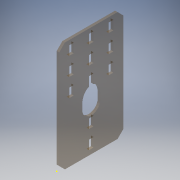
# Autodesk Inventor part: Sleigh
Saved by Autodesk Inventor 2019 (Build 230136000, 136)
## iProperties
Created: 2019-01-14
Part Number: Sleigh
Material: Polycarbonate, Smoke
Document SubType Name: Modeling
Designer: nxgam
Density: 1.2 g/cm^3
Appearance: Polycarbonate - Smoked
Author: nxgam
Autodesk Inventor part; units mm, degrees
ref_plane "YZ Plane" through (0, 0, 0) normal (1, 0, 0) x (0, 1, 0)
ref_plane "XZ Plane" through (0, 0, 0) normal (0, 1, 0) x (-1, 0, 0)
ref_plane "XY Plane" through (0, 0, 0) normal (0, 0, 1) x (1, 0, 0)
sketch "Sketch1" plane through (0, 0, 0) normal (1, 0, 0) x (0, 1, 0)
  line L0 (0, 0) -> (121.92, 0)
  line L1 (121.92, 0) -> (121.92, -71.12)
  line L2 (121.92, -71.12) -> (0, -71.12)
  line L3 (0, -71.12) -> (0, 0)
  dimension "d0" = 121.92
  dimension "d1" = 71.12
  constraints: 8 end point, 2 parallel, 1 horizontal, 1 perpendicular
  measures "d0" distance of L1.end L2.end
  measures "d1" distance of L0.end L1.end
extrude "Extrusion1" add sketch "Sketch1" along normal blind 2.794
sketch "Sketch2" plane through (2.794, 0, 0) normal (1, 0, 0) x (0, 0, -1)
  line L0 (0, 121.92) -> (0, 0) projected
  line L1 (0, 0) -> (71.12, 0) projected
  line L2 (71.12, 0) -> (71.12, 121.92) projected
  line L3 (71.12, 121.92) -> (0, 121.92) projected
  line L4 (71.12, 121.92) -> (0, 121.92) construction
  line L5 (35.56, 121.92) -> (35.56, 0) construction
  line L6 (33.02, 5.08) -> (38.1, 5.08)
  line L7 (38.1, 5.08) -> (38.1, 15.24)
  line L8 (38.1, 15.24) -> (33.02, 15.24)
  line L9 (33.02, 15.24) -> (33.02, 5.08)
  line L10 (33.02, 25.4) -> (38.1, 25.4)
  line L11 (38.1, 25.4) -> (38.1, 35.56)
  line L12 (38.1, 35.56) -> (33.02, 35.56)
  line L13 (33.02, 35.56) -> (33.02, 25.4)
  line L14 (33.02, 45.72) -> (38.1, 45.72)
  line L15 (38.1, 45.72) -> (38.1, 55.88)
  line L16 (38.1, 55.88) -> (33.02, 55.88)
  line L17 (33.02, 55.88) -> (33.02, 45.72)
  line L18 (33.02, 66.04) -> (38.1, 66.04)
  line L19 (38.1, 66.04) -> (38.1, 76.2)
  line L20 (38.1, 76.2) -> (33.02, 76.2)
  line L21 (33.02, 76.2) -> (33.02, 66.04)
  line L22 (33.02, 86.36) -> (38.1, 86.36)
  line L23 (38.1, 86.36) -> (38.1, 96.52)
  line L24 (38.1, 96.52) -> (33.02, 96.52)
  line L25 (33.02, 96.52) -> (33.02, 86.36)
  line L26 (33.02, 106.68) -> (38.1, 106.68)
  line L27 (38.1, 106.68) -> (38.1, 116.84)
  line L28 (38.1, 116.84) -> (33.02, 116.84)
  line L29 (33.02, 116.84) -> (33.02, 106.68)
  line L30 (11.049, 86.36) -> (16.129, 86.36)
  line L31 (16.129, 86.36) -> (16.129, 96.52)
  line L32 (11.049, 96.52) -> (11.049, 86.36)
  line L33 (16.129, 96.52) -> (11.049, 96.52)
  line L34 (11.049, 106.68) -> (16.129, 106.68)
  line L35 (11.049, 116.84) -> (11.049, 106.68)
  line L36 (16.129, 106.68) -> (16.129, 116.84)
  line L37 (16.129, 116.84) -> (11.049, 116.84)
  line L38 (11.049, 66.04) -> (16.129, 66.04)
  line L39 (11.049, 76.2) -> (11.049, 66.04)
  line L40 (16.129, 66.04) -> (16.129, 76.2)
  line L41 (16.129, 76.2) -> (11.049, 76.2)
  line L42 (54.991, 86.36) -> (60.071, 86.36)
  line L43 (60.071, 86.36) -> (60.071, 96.52)
  line L44 (54.991, 96.52) -> (54.991, 86.36)
  line L45 (60.071, 96.52) -> (54.991, 96.52)
  line L46 (54.991, 106.68) -> (60.071, 106.68)
  line L47 (54.991, 116.84) -> (54.991, 106.68)
  line L48 (60.071, 106.68) -> (60.071, 116.84)
  line L49 (60.071, 116.84) -> (54.991, 116.84)
  line L50 (54.991, 66.04) -> (60.071, 66.04)
  line L51 (54.991, 76.2) -> (54.991, 66.04)
  line L52 (60.071, 66.04) -> (60.071, 76.2)
  line L53 (60.071, 76.2) -> (54.991, 76.2)
  line L54 (33.02, 86.36) -> (38.1, 86.36)
  line L55 (38.1, 86.36) -> (38.1, 96.52)
  line L56 (33.02, 96.52) -> (33.02, 86.36)
  line L57 (38.1, 96.52) -> (33.02, 96.52)
  line L58 (33.02, 106.68) -> (38.1, 106.68)
  line L59 (33.02, 116.84) -> (33.02, 106.68)
  line L60 (38.1, 106.68) -> (38.1, 116.84)
  line L61 (38.1, 116.84) -> (33.02, 116.84)
  line L62 (33.02, 66.04) -> (38.1, 66.04)
  line L63 (33.02, 76.2) -> (33.02, 66.04)
  line L64 (38.1, 66.04) -> (38.1, 76.2)
  line L65 (38.1, 76.2) -> (33.02, 76.2)
  point P0 (35.56, 15.24)
  point P1 (35.56, 35.56)
  point P2 (35.56, 55.88)
  point P3 (35.56, 76.2)
  point P4 (35.56, 96.52)
  point P5 (35.56, 116.84)
  point P6 (13.589, 96.52)
  point P7 (13.589, 116.84)
  point P8 (13.589, 76.2)
  point P9 (57.531, 96.52)
  point P10 (57.531, 116.84)
  point P11 (57.531, 76.2)
  point P12 (35.56, 96.52)
  point P13 (35.56, 116.84)
  point P14 (35.56, 76.2)
  dimension "d4" = 5.08
  dimension "d5" = 10.16
  dimension "d6" = 5.08
  dimension "d9" = 20.32
  dimension "d18" = 21.971
  dimension "d21" = 21.971
  constraints: 122 end point, 3 horizontal, 3 midpoint, 2 parallel, 1 perpendicular, 1 point on line, 1 vertical, 126 other
  measures "d4" distance of L7.end L8.end
  measures "d5" distance of L6.end L7.end
  measures "d6" distance between parallel lines of L6 L1
  measures "d9" distance of L6.start L10.start
  measures "d18" distance of L22.start L30.start
  measures "d21" distance of L22.start L42.start
extrude "Extrusion2" cut sketch "Sketch2" against normal blind 25.4 contours L3 L2 L1 L0 | L32 L33 L31 L30 | L35 L37 L36 L34 | L39 L41 L40 L38 | L44 L45 L43 L42 | L47 L49 L48 L46 | L51 L53 L52 L50 keep common part
extrude "Extrusion3" cut sketch "Sketch2" against normal blind 25.4 keep common part
sketch "Sketch3" plane through (2.794, 0, 0) normal (1, 0, 0) x (0, 0, -1)
  ellipse E0 centre (35.56, 53.0414) end of major axis (35.56, 41.2576) minor radius 8.332 (40.2212, 62.8087) -> (30.9261, 62.8347) ccw construction
  spline S0 degree 3 poles (30.9261, 62.8347) (30.9327, 62.8286) (30.9386, 62.8221) (30.9557, 62.8007) (30.9663, 62.7802) (30.977, 62.7425) (30.9787, 62.7187) (30.9751, 62.672) (30.9665, 62.6409) (30.9201, 62.5239) (30.844, 62.4329) (30.6139, 62.201) (30.3871, 62.0485) (30.1451, 61.9341) (30.1067, 61.9173) (30.0669, 61.9017) knots 0.147565 0.147565 0.147565 0.147565 0.150034 0.150034 0.1558 0.1558 0.161773 0.161773 0.169845 0.169845 0.199517 0.199517 0.267842 0.267842 0.279835 0.279835 0.279835 0.279835 construction
  ellipse E1 centre (35.56, 53.0414) end of major axis (35.56, 41.2576) minor radius 8.332 (30.0669, 61.9017) -> (27.23, 53.3005) ccw construction
  spline S1 degree 3 poles (27.23, 53.3005) (27.2588, 53.2719) (27.2851, 53.2407) (27.334, 53.1732) (27.3565, 53.1364) (27.3764, 53.0984) knots -0.025032 -0.025032 -0.025032 -0.025032 -0.012859 -0.012859 0 0 0 0 construction
  spline S2 degree 3 poles (27.3764, 53.0984) (27.3563, 53.0613) (27.3336, 53.0254) (27.2841, 52.9599) (27.2576, 52.9297) (27.2286, 52.9024) knots -0.024627 -0.024627 -0.024627 -0.024627 -0.011976 -0.011976 -0.000005 -0.000005 -0.000005 -0.000005 construction
  ellipse E2 centre (35.56, 53.0414) end of major axis (35.56, 41.2576) minor radius 8.332 (27.2286, 52.9024) -> (27.2377, 52.473) ccw construction
  spline S3 degree 3 poles (27.2377, 52.473) (27.2678, 52.4474) (27.2955, 52.4189) (27.3478, 52.3562) (27.372, 52.3217) (27.3937, 52.2857) knots -0.024476 -0.024476 -0.024476 -0.024476 -0.012604 -0.012604 0 0 0 0 construction
  spline S4 degree 3 poles (27.3937, 52.2857) (27.3755, 52.2465) (27.3546, 52.2085) (27.3086, 52.1382) (27.2836, 52.1055) (27.256, 52.0754) knots -0.025198 -0.025198 -0.025198 -0.025198 -0.012267 -0.012267 -0.000005 -0.000005 -0.000005 -0.000005 construction
  ellipse E3 centre (35.56, 53.0414) end of major axis (35.56, 41.2576) minor radius 8.332 (27.256, 52.0754) -> (39.4571, 42.626) ccw construction
  spline S5 degree 3 poles (39.4571, 42.626) (39.4604, 42.6731) (39.4664, 42.7203) (39.4838, 42.8124) (39.4952, 42.8577) (39.5094, 42.902) knots -0.028123 -0.028123 -0.028123 -0.028123 -0.013949 -0.013949 0 0 0 0 construction
  spline S6 degree 3 poles (39.5094, 42.902) (39.5437, 42.8955) (39.577, 42.8851) (39.6424, 42.8569) (39.674, 42.839) (39.7037, 42.8182) knots -0.021367 -0.021367 -0.021367 -0.021367 -0.01089 -0.01089 -0.00001 -0.00001 -0.00001 -0.00001 construction
  ellipse E4 centre (35.56, 53.0414) end of major axis (35.56, 41.2576) minor radius 8.332 (39.7037, 42.8182) -> (39.9645, 43.0386) ccw construction
  spline S7 degree 3 poles (39.9645, 43.0386) (39.9654, 43.0862) (39.9691, 43.1338) (39.9819, 43.2275) (39.991, 43.274) (40.0029, 43.3195) knots -0.02838 -0.02838 -0.02838 -0.02838 -0.014121 -0.014121 0 0 0 0 construction
  spline S8 degree 3 poles (40.0029, 43.3195) (40.0373, 43.3164) (40.0711, 43.3093) (40.1378, 43.2875) (40.1703, 43.2728) (40.2011, 43.2549) knots -0.021052 -0.021052 -0.021052 -0.021052 -0.010689 -0.010689 -0.000009 -0.000009 -0.000009 -0.000009 construction
  ellipse E5 centre (35.56, 53.0414) end of major axis (35.56, 41.2576) minor radius 8.332 (40.2011, 43.2549) -> (41.1095, 61.8311) ccw construction
  spline S9 degree 3 poles (41.1095, 61.8311) (41.0496, 61.8526) (40.9919, 61.8776) (40.734, 62.0024) (40.5086, 62.1569) (40.2806, 62.3908) (40.2052, 62.4825) (40.1599, 62.5999) (40.1516, 62.6311) (40.1484, 62.6778) (40.1503, 62.7016) (40.1613, 62.7392) (40.1721, 62.7596) (40.1941, 62.7867) (40.2073, 62.7989) (40.2212, 62.8087) knots 0.103426 0.103426 0.103426 0.103426 0.121046 0.121046 0.189371 0.189371 0.219043 0.219043 0.227115 0.227115 0.233088 0.233088 0.238854 0.238854 0.243583 0.243583 0.243583 0.243583 construction
  ellipse E6 centre (35.56, 53.0524) end of major axis (35.56, 40.1371) minor radius 9.1321 construction
  ellipse E7 centre (35.56, 52.9268) end of major axis (35.56, 42.9637) minor radius 7.045 (39.5734, 61.1151) -> (37.2879, 62.5856) ccw construction
  line L0 (37.2879, 62.5856) -> (37.0953, 61.1151) construction
  line L1 (37.0953, 61.1151) -> (39.5734, 61.1151) construction
  line L2 (29.0123, 59.6726) -> (28.7127, 59.6726) construction
  ellipse E8 centre (35.56, 52.9268) end of major axis (35.56, 41.1252) minor radius 8.345 (42.4073, 59.6726) -> (28.7127, 59.6726) ccw construction
  line L3 (42.4073, 59.6726) -> (42.1077, 59.6726) construction
  ellipse E9 centre (35.56, 52.9268) end of major axis (35.56, 64.3833) minor radius 8.101 (42.4504, 58.9514) -> (42.1077, 59.6726) ccw construction
  line L4 (42.4504, 58.9514) -> (36.9155, 58.9514) construction
  line L5 (36.9155, 58.9514) -> (37.0257, 59.6726) construction
  line L6 (37.0257, 59.6726) -> (36.1561, 59.6726) construction
  line L7 (36.1561, 59.6726) -> (36.0459, 58.9514) construction
  line L8 (36.0459, 58.9514) -> (33.4082, 58.9514) construction
  line L9 (33.4082, 58.9514) -> (33.9116, 57.9159) construction
  line L10 (33.9116, 57.9159) -> (33.2456, 57.2685) construction
  line L11 (33.2456, 57.2685) -> (32.7453, 57.1196) construction
  line L12 (32.7453, 57.1196) -> (31.855, 58.9514) construction
  line L13 (31.855, 58.9514) -> (28.6696, 58.9514) construction
  ellipse E10 centre (35.56, 52.9268) end of major axis (35.56, 64.3833) minor radius 8.101 (29.0123, 59.6726) -> (28.6696, 58.9514) ccw construction
  line L14 (32.132, 61.1151) -> (36.1698, 61.1151) construction
  line L15 (36.1698, 61.1151) -> (36.3931, 62.82) construction
  ellipse E11 centre (35.56, 52.9268) end of major axis (35.56, 42.9637) minor radius 7.045 (36.3931, 62.82) -> (31.9524, 61.4845) ccw construction
  line L16 (31.9524, 61.4845) -> (32.132, 61.1151) construction
  line L17 (38.6371, 57.0165) -> (40.2416, 58.5764) construction
  line L18 (40.2416, 58.5764) -> (40.9667, 57.0846) construction
  line L19 (40.9667, 57.0846) -> (40.1513, 56.2919) construction
  line L20 (40.1513, 56.2919) -> (38.6371, 57.0165) construction
  line L21 (38.6371, 57.0165) -> (40.1513, 56.2919) construction
  line L22 (40.1513, 56.2919) -> (40.9667, 57.0846) construction
  line L23 (40.9667, 57.0846) -> (40.7011, 57.631) construction
  line L24 (40.7011, 57.631) -> (41.0218, 57.631) construction
  ellipse E12 centre (35.56, 52.9268) end of major axis (35.56, 43.8829) minor radius 6.395 (30.0982, 57.631) -> (41.0218, 57.631) ccw construction
  line L25 (30.0982, 57.631) -> (32.4968, 57.631) construction
  line L26 (32.4968, 57.631) -> (32.7453, 57.1196) construction
  line L27 (32.7453, 57.1196) -> (33.2456, 57.2685) construction
  line L28 (33.2456, 57.2685) -> (33.6185, 57.631) construction
  line L29 (33.6185, 57.631) -> (39.2691, 57.631) construction
  line L30 (39.2691, 57.631) -> (38.6371, 57.0165) construction
  ellipse E13 centre (35.56, 53.0524) end of major axis (35.56, 39.5904) minor radius 9.983
  point P0 (0, 0)
  dimension "d26" = 13.462
  constraints: 62 end point, 11 horizontal, 161 other
extrude "Extrusion4" cut sketch "Sketch3" against normal blind 25.4
sketch "Sketch4" plane through (0, 0, 0) normal (-1, 0, 0) x (0, 0, 1)
  point P0 (0, 0)
sketch "Sketch5" plane through (0, 0, 0) normal (-1, 0, 0) x (0, 0, 1)
  ellipse E0 centre (-35.56, 53.0524) end of major axis (-35.56, 66.5144) minor radius 9.983 (-38.1, 66.0713) -> (-33.02, 66.0713) ccw projected
  line L0 (-38.1, 76.2) -> (-38.1, 66.0713) projected
  line L1 (-33.02, 76.2) -> (-38.1, 76.2) projected
  line L2 (-33.02, 66.0713) -> (-33.02, 76.2) projected
  line L3 (-60.071, 76.2) -> (-60.071, 66.04) projected
  line L4 (-54.991, 76.2) -> (-60.071, 76.2) projected
  line L5 (-54.991, 66.04) -> (-54.991, 76.2) projected
  line L6 (-60.071, 66.04) -> (-54.991, 66.04) projected
  line L7 (-60.071, 116.84) -> (-60.071, 106.68) projected
  line L8 (-54.991, 116.84) -> (-60.071, 116.84) projected
  line L9 (-54.991, 106.68) -> (-54.991, 116.84) projected
  line L10 (-60.071, 106.68) -> (-54.991, 106.68) projected
  line L11 (-60.071, 96.52) -> (-60.071, 86.36) projected
  line L12 (-54.991, 96.52) -> (-60.071, 96.52) projected
  line L13 (-54.991, 86.36) -> (-54.991, 96.52) projected
  line L14 (-60.071, 86.36) -> (-54.991, 86.36) projected
  line L15 (-16.129, 76.2) -> (-16.129, 66.04) projected
  line L16 (-11.049, 76.2) -> (-16.129, 76.2) projected
  line L17 (-11.049, 66.04) -> (-11.049, 76.2) projected
  line L18 (-16.129, 66.04) -> (-11.049, 66.04) projected
  line L19 (-16.129, 116.84) -> (-16.129, 106.68) projected
  line L20 (-11.049, 116.84) -> (-16.129, 116.84) projected
  line L21 (-11.049, 106.68) -> (-11.049, 116.84) projected
  line L22 (-16.129, 106.68) -> (-11.049, 106.68) projected
  line L23 (-16.129, 96.52) -> (-16.129, 86.36) projected
  line L24 (-11.049, 96.52) -> (-16.129, 96.52) projected
  line L25 (-11.049, 86.36) -> (-11.049, 96.52) projected
  line L26 (-16.129, 86.36) -> (-11.049, 86.36) projected
  line L27 (-38.1, 116.84) -> (-38.1, 106.68) projected
  line L28 (-33.02, 116.84) -> (-38.1, 116.84) projected
  line L29 (-33.02, 106.68) -> (-33.02, 116.84) projected
  line L30 (-38.1, 106.68) -> (-33.02, 106.68) projected
  line L31 (-38.1, 96.52) -> (-38.1, 86.36) projected
  line L32 (-33.02, 96.52) -> (-38.1, 96.52) projected
  line L33 (-33.02, 86.36) -> (-33.02, 96.52) projected
  line L34 (-38.1, 86.36) -> (-33.02, 86.36) projected
  line L35 (-38.1, 35.56) -> (-38.1, 25.4) projected
  line L36 (-33.02, 35.56) -> (-38.1, 35.56) projected
  line L37 (-33.02, 25.4) -> (-33.02, 35.56) projected
  line L38 (-38.1, 25.4) -> (-33.02, 25.4) projected
  line L39 (-38.1, 15.24) -> (-38.1, 5.08) projected
  line L40 (-33.02, 15.24) -> (-38.1, 15.24) projected
  line L41 (-33.02, 5.08) -> (-33.02, 15.24) projected
  line L42 (-38.1, 5.08) -> (-33.02, 5.08) projected
  line L43 (0, 0) -> (0, 121.92) projected
  line L44 (0, 121.92) -> (-71.12, 121.92) projected
  line L45 (-71.12, 121.92) -> (-71.12, 0) projected
  line L46 (-71.12, 0) -> (0, 0) projected
  line L47 (-25.577, 53.0524) -> (-25.577, 47.2295)
  ellipse E1 centre (-35.56, 53.0524) end of major axis (-35.56, 66.5144) minor radius 9.983 (-38.1, 66.0713) -> (-33.02, 66.0713) ccw projected
  line L48 (-45.543, 53.0524) -> (-45.543, 47.2295)
  line L49 (-45.543, 47.2295) -> (-25.577, 47.2295) construction
  arc A0 (-45.543, 47.2295) -> (-25.577, 47.2295) centre (-35.56, 47.2295) ccw
  line L50 (-25.577, 53.0524) -> (-45.543, 53.0524)
  constraints: 8 end point, 5 vertical, 2 horizontal, 2 point on circle, 2 tangent, 1 centre point, 4 other
extrude "Extrusion5" cut sketch "Sketch5" against normal blind 25.4 contours L50 E0 | E0 L47 A0 L48
chamfer "Chamfer1" distance 6.35 angle 45 4 edges at (1.397, 121.92, -71.12) (1.397, 121.92, 0) (1.397, 0, 0) (1.397, 0, -71.12)
equation "\"d9\" = 2 * d5"
body "Solid1"
